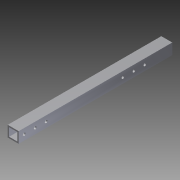
# Autodesk Inventor part: 10 inch side piece
Saved by Autodesk Inventor 2011 SP1 (Build 150282100, 282)
## iProperties
Created: 2012-01-20
Part Number: 10 inch side piece
Document SubType Name: Modeling
Designer: Christopher
Density: 1 g/cm^3
Author: Christopher
Autodesk Inventor part; units mm, degrees
ref_plane "YZ Plane" through (0, 0, 0) normal (1, 0, 0) x (0, 1, 0)
ref_plane "XZ Plane" through (0, 0, 0) normal (0, 1, 0) x (-1, 0, 0)
ref_plane "XY Plane" through (0, 0, 0) normal (0, 0, 1) x (1, 0, 0)
sketch "Sketch1" plane through (0, 0, 0) normal (0, 0, 1) x (1, 0, 0)
  line L0 (0, 0) -> (25.4, 0)
  line L1 (25.4, 0) -> (25.4, 25.4)
  line L2 (25.4, 25.4) -> (0, 25.4)
  line L3 (0, 25.4) -> (0, 0)
  line L4 (3.175, 22.225) -> (22.225, 22.225)
  line L5 (22.225, 22.225) -> (22.225, 3.175)
  line L6 (22.225, 3.175) -> (3.175, 3.175)
  line L7 (3.175, 3.175) -> (3.175, 22.225)
  dimension "d0" = 25.4
  dimension "d1" = 25.4
  dimension "d2" = 3.175
  constraints: 16 end point, 4 parallel, 2 perpendicular, 1 horizontal, 3 other
  measures "d0" distance of L1.end L2.end
  measures "d1" distance of L2.end L0.start
  measures "d2" distance between parallel lines of L3 L7
extrude "Extrusion1" add sketch "Sketch1" against normal blind 355.6
sketch "Sketch2" plane through (0, 0, 0) normal (-1, 0, 0) x (0, 0, 1)
  line L0 (-355.6, 25.4) -> (-355.6, 0) projected
  line L1 (0, 25.4) -> (0, 0) projected
  point P0 (-266.7, 12.7)
  point P1 (-241.3, 12.7)
  point P2 (-215.9, 12.7)
  point P3 (-12.7, 12.7)
  point P4 (-38.1, 12.7)
  point P5 (-63.5, 12.7)
  dimension "d5" = 88.9
  dimension "d6" = 25.4
  dimension "d7" = 25.4
  dimension "d8" = 25.4
  dimension "d9" = 25.4
  dimension "d10" = 12.7
  measures "d5" distance from line of L0 point (-266.7, 12.7)
  measures "d6" distance of point (-241.3, 12.7) point (-215.9, 12.7)
  measures "d7" distance of point (-266.7, 12.7) point (-241.3, 12.7)
  measures "d8" distance of point (-63.5, 12.7) point (-38.1, 12.7)
  measures "d9" distance of point (-38.1, 12.7) point (-12.7, 12.7)
  measures "d10" distance from line of L1 point (-12.7, 12.7)
hole "Hole1" at (0, 12.7, -266.7) at (0, 12.7, -241.3) at (0, 12.7, -215.9) at (0, 12.7, -12.7) at (0, 12.7, -38.1) at (0, 12.7, -63.5) direction (1, 0, 0) diameter 6.35 depth 25.4 tip angle 118
sketch "Sketch3" plane through (0, 25.4, 0) normal (0, 1, 0) x (1, 0, 0)
  line L0 (25.4, 355.6) -> (0, 355.6) projected
  point P0 (12.7, 342.9)
  point P1 (12.7, 317.5)
  point P2 (12.7, 292.1)
  dimension "d18" = 25.4
  dimension "d19" = 25.4
  dimension "d20" = 12.7
  measures "d18" distance of point (12.7, 292.1) point (12.7, 317.5)
  measures "d19" distance of point (12.7, 342.9) point (12.7, 317.5)
  measures "d20" distance from line of L0 point (12.7, 342.9)
hole "Hole2" at (12.7, 25.4, -342.9) at (12.7, 25.4, -317.5) at (12.7, 25.4, -292.1) direction (0, -1, 0) diameter 6.35 depth 25.4 tip angle 118
body "Solid1"
